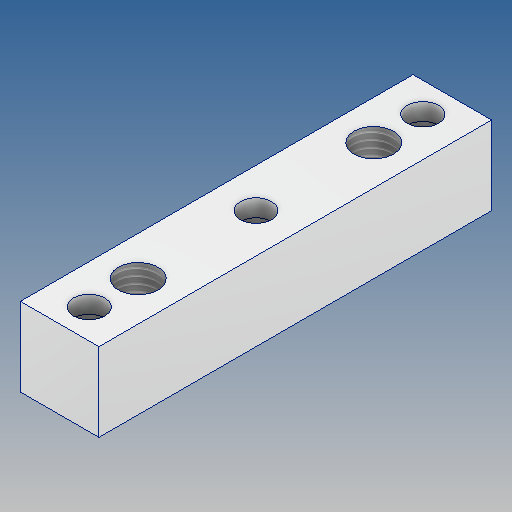
# Autodesk Inventor part: 106.014.01_Anbindung_Vereinzelung
Saved by Autodesk Inventor 2021 (Build 250183000, 183)
## iProperties
Created: 2021-11-26
Part Number: 106.014.01_Anbindung_Vereinzelung
Material: Aluminium 6061
Document SubType Name: Modeling
Designer: Oliver Ungerer
Density: 2.7 g/cm^3
Appearance: Aluminium - flach
Mass: 98.1429 g
Surface Area: 105.897 cm^2
Volume: 36.3492 cm^3
Author: Oliver Ungerer
Title: Befestigungskonsole
Autodesk Inventor part; units mm, degrees
ref_plane "YZ Plane" through (0, 0, 0) normal (1, 0, 0) x (0, 1, 0)
ref_plane "XZ Plane" through (0, 0, 0) normal (0, 1, 0) x (-1, 0, 0)
ref_plane "XY Plane" through (0, 0, 0) normal (0, 0, 1) x (1, 0, 0)
sketch "Skizze1" plane through (0, 0, 0) normal (0, 1, 0) x (-1, 0, 0)
  line L0 (10, 50) -> (-10, 50)
  line L1 (-10, 50) -> (-10, -50)
  line L2 (-10, -50) -> (10, -50)
  line L3 (10, -50) -> (10, 50)
  line L4 (10, 50) -> (-10, -50) construction
  line L5 (-10, 50) -> (10, -50) construction
  point P0 (0, 0)
  dimension "d0" = 100
  dimension "d1" = 20
  constraints: 12 end point, 2 midpoint, 2 parallel, 1 horizontal, 1 perpendicular
  measures "d0" distance between parallel lines of L2 L0
  measures "d1" distance between parallel lines of L1 L3
extrude "Extrusion1" add sketch "Skizze1" along normal mid plane 20
sketch "Skizze2" plane through (0, 10, 0) normal (0, 1, 0) x (1, 0, 0)
  line L0 (-10, 50) -> (-10, -50) projected
  line L1 (-10, 0) -> (10, 0)
  line L2 (10, -50) -> (10, 50) projected
  point P0 (0, 0)
  point P1 (0, -30)
  point P2 (0, 30)
  dimension "d4" = 60
  constraints: 2 end point, 2 midpoint, 1 symmetric about line
  measures "d4" distance of point (0, -30) point (0, 30)
hole "Bohrung1" at (0, 10, 30) at (0, 10, -30) direction (0, -1, 0) diameter 10.106 depth 12 tip angle 118 thread size "M12x1.75" class "6H" standard "ISO Metric profile"
sketch "Skizze3" plane through (0, 10, 0) normal (0, 1, 0) x (1, 0, 0)
  circle A0 centre (0, -30) radius 5.053 projected
  point P0 (0, 0)
  constraints: 1 coincident
hole "Bohrung2" at (0, 10, 30) direction (0, -1, 0) diameter 4.134 end through all thread size "M5x0.8" class "6H" standard "ISO Metric profile"
sketch "Skizze4" plane through (0, 10, 0) normal (0, 1, 0) x (1, 0, 0)
  circle A0 centre (0, 30) radius 5.053 projected
  point P0 (0, 0)
  constraints: 1 coincident
hole "Bohrung3" at (0, 10, -30) direction (0, -1, 0) diameter 4.134 end through all thread size "M5x0.8" class "6H" standard "ISO Metric profile"
sketch "Skizze5" plane through (0, 10, 0) normal (0, 1, 0) x (1, 0, 0)
  line L0 (-10, -50) -> (-10, 50) projected
  line L1 (-10, 0) -> (10, 0)
  line L2 (10, 50) -> (10, -50) projected
  point P0 (0, 0)
  point P1 (0, -42.5)
  point P2 (0, 0)
  point P3 (0, 42.5)
  point P4 (0, 0)
  dimension "d26" = 85
  constraints: 2 coincident, 2 end point, 2 midpoint, 1 symmetric about line
  measures "d26" distance of point (0, 42.5) point (0, -42.5)
hole "Bohrung4" at (0, 10, 0) at (0, 10, -42.5) at (0, 10, 42.5) direction (0, -1, 0) diameter 4.5 depth 20 counterbore diameter 8 counterbore depth 4.4
